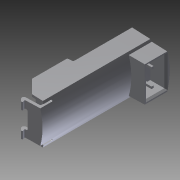
# Autodesk Inventor part: 566716
Saved by Autodesk Inventor 2014 (Build 180170000, 170)
## iProperties
Category: Pneumatics
Company: Autodesk Inc.
Created: 2013-12-30
Part Number: 566716
Catalog Web Link: http://www.festo.com/rep/ko_kr/assets/pdf/VUVG_KR_new.pdf
Vendor: FESTO
Document SubType Name: Modeling
Designer: Autodesk Inc.
Manufacturer: FESTO
Density: 1 g/cm^3
Material: Generic
Appearance: RGB(175.94999939203154,175.94999939203154,175.94999939203154)
Title: 566716 VAVE-L1-1H2-LR
Author: Autodesk Inc.
Autodesk Inventor part; units mm, degrees
sketch "Sketch_23" plane through (0, 0, 0) normal (0, 0, 1) x (1, 0, 0)
  line L0 (-6.5, 4.0058) -> (-3.404, 0.9098)
  line L1 (-3.404, 0.9098) -> (-2.55, 0.8949)
  line L2 (-2.55, 0.8949) -> (-2.55, 0.5951)
  line L3 (-2.55, 0.5951) -> (-4.4413, 0.5621)
  arc A0 (-4.4413, 0.5621) -> (-4.8099, -0.2659) centre (-4.4326, 0.0622) ccw
  line L4 (-4.8099, -0.2659) -> (-4.3557, -0.7885)
  arc A1 (-4.3557, -0.7885) -> (-4.1395, -0.8847) centre (-4.1443, -0.6048) ccw
  line L5 (-4.1395, -0.8847) -> (-3.9988, -0.8823)
  arc A2 (-3.9988, -0.8823) -> (-3.9044, -0.7547) centre (-4.0006, -0.7823) ccw
  line L6 (-3.9044, -0.7547) -> (-4.0447, -0.2655)
  arc A3 (-3.9521, -0.138) -> (-4.0447, -0.2655) centre (-3.9486, -0.2379) ccw
  line L7 (-3.9521, -0.138) -> (0, 0)
  line L8 (0, 0) -> (0, 29)
  line L9 (0, 29) -> (-5.2, 29)
  line L10 (-5.2, 29) -> (-5.2, 15.3866)
  arc A4 (-5.4739, 15.0878) -> (-5.2, 15.3866) centre (-5.5, 15.3866) ccw
  line L11 (-5.4739, 15.0878) -> (-6.2261, 15.022)
  arc A5 (-6.2261, 15.022) -> (-6.5, 14.7231) centre (-6.2, 14.7231) ccw
  line L12 (-6.5, 14.7231) -> (-6.5, 4.0058)
  constraints: 26 end point, 12 point on circle, 6 centre point
extrude "Extrusion1" add sketch "Sketch_23" along normal mid plane 10
sketch "Sketch_1" plane through (0, -5, 0) normal (0, 1, 0) x (1, 0, 0)
  line L0 (-7, 10) -> (-7, -10)
  line L1 (-7, -10) -> (5, -10)
  line L2 (5, -10) -> (5, 10)
  line L3 (5, 10) -> (-7, 10)
  line L4 (-6.5, 4.934) -> (-6.5, -4.934)
  line L5 (-6.5, -4.934) -> (-0.7835, -4.7843)
  arc A0 (-0.7835, -4.7843) -> (-0.7835, 4.7843) centre (-15, 0) ccw
  line L6 (-0.7835, 4.7843) -> (-6.5, 4.934)
  constraints: 14 end point, 2 point on circle, 1 centre point
sketch "Sketch_3" plane through (0, 0, 0) normal (1, 0, 0) x (0, 1, 0)
  line L0 (-3, 5) -> (-3, -5)
  line L1 (-3, -5) -> (1.164, -5)
  line L2 (1.164, -5) -> (1.164, -4.23)
  line L3 (1.164, -4.23) -> (2.722, -4.23)
  arc A0 (2.722, -4.23) -> (2.722, -3.851) centre (2.722, -4.0405) ccw
  line L4 (2.722, -3.851) -> (-1, -3.851)
  line L5 (-1, -3.851) -> (-1, -2.1245)
  line L6 (-1, -2.1245) -> (-0.9, -2.1245)
  line L7 (-0.9, -2.1245) -> (-0.9, 2.1245)
  line L8 (-0.9, 2.1245) -> (-1, 2.1245)
  line L9 (-1, 2.1245) -> (-1, 3.851)
  line L10 (-1, 3.851) -> (2.722, 3.851)
  arc A1 (2.722, 3.851) -> (2.722, 4.23) centre (2.722, 4.0405) ccw
  line L11 (2.722, 4.23) -> (1.164, 4.23)
  line L12 (1.164, 4.23) -> (1.164, 5)
  line L13 (1.164, 5) -> (-3, 5)
  constraints: 28 end point, 4 point on circle, 2 centre point
sketch "Sketch_4" plane through (0, 0, 0) normal (0, 1, 0) x (-1, 0, 0)
  line L0 (6.4, -2.2572) -> (6.4, 2.2572)
  line L1 (6.4, 2.2572) -> (3.6843, 2.1149)
  arc A0 (3.6843, 2.1149) -> (3.4, 1.8153) centre (3.7, 1.8153) ccw
  line L2 (3.4, 1.8153) -> (3.4, -1.8153)
  arc A1 (3.4, -1.8153) -> (3.6843, -2.1149) centre (3.7, -1.8153) ccw
  line L3 (3.6843, -2.1149) -> (6.4, -2.2572)
  constraints: 8 end point, 4 point on circle, 2 centre point
extrude "Extrusion2" cut sketch "Sketch_4" along normal mid plane 2
sketch "Sketch_5" plane through (0, 0, 0) normal (0, 0, 1) x (1, 0, 0)
  line L0 (-15, 0.1264) -> (-15, 3.912)
  line L1 (-15, 3.912) -> (-0.55, 3.912)
  line L2 (-0.55, 3.912) -> (-0.55, 0.9207)
  arc A0 (-0.8395, 0.6209) -> (-0.55, 0.9207) centre (-0.85, 0.9207) ccw
  line L3 (-0.8395, 0.6209) -> (-15, 0.1264)
  line L4 (-15, 0.1264) -> (-15, 3.912)
  constraints: 10 end point, 2 point on circle, 1 centre point
revolve "Revolution1" cut sketch "Sketch_5" angle 60 mid plane about axis through (-15, 0.1264, 0) along (0, 1, 0)
sketch "Sketch_6" plane through (0, 0, 5) normal (0, 0, 1) x (1, 0, 0)
  line L0 (-6.5, 4.0058) -> (-3.404, 0.9098)
  line L1 (-3.404, 0.9098) -> (0, 0.8504)
  line L2 (0, 0.8504) -> (0, 27.33)
  line L3 (0, 27.33) -> (-5.2, 27.33)
  line L4 (-5.2, 27.33) -> (-5.2, 15.3866)
  arc A0 (-5.4739, 15.0878) -> (-5.2, 15.3866) centre (-5.5, 15.3866) ccw
  line L5 (-5.4739, 15.0878) -> (-6.2261, 15.022)
  arc A1 (-6.2261, 15.022) -> (-6.5, 14.7231) centre (-6.2, 14.7231) ccw
  line L6 (-6.5, 14.7231) -> (-6.5, 4.0058)
  constraints: 14 end point, 4 point on circle, 2 centre point
sketch "Sketch_7" plane through (0, 0, -5) normal (0, 0, 1) x (1, 0, 0)
  line L0 (-6.5, 4.0058) -> (-3.404, 0.9098)
  line L1 (-3.404, 0.9098) -> (0, 0.8504)
  line L2 (0, 0.8504) -> (0, 27.33)
  line L3 (0, 27.33) -> (-5.2, 27.33)
  line L4 (-5.2, 27.33) -> (-5.2, 15.3866)
  arc A0 (-5.4739, 15.0878) -> (-5.2, 15.3866) centre (-5.5, 15.3866) ccw
  line L5 (-5.4739, 15.0878) -> (-6.2261, 15.022)
  arc A1 (-6.2261, 15.022) -> (-6.5, 14.7231) centre (-6.2, 14.7231) ccw
  line L6 (-6.5, 14.7231) -> (-6.5, 4.0058)
  constraints: 14 end point, 4 point on circle, 2 centre point
extrude "Extrusion3" cut sketch "Sketch_3" against normal blind 7
extrude "Extrusion4" add sketch "Sketch_6" against normal blind 0.77
extrude "Extrusion5" add sketch "Sketch_7" along normal blind 0.77
sketch "Sketch_12" plane through (0, 0.85, 0) normal (0, 1, 0) x (1, 0, 0)
  line L0 (-6.5, 4.384) -> (-6.5, -4.384)
  line L1 (-6.5, -4.384) -> (-1.2087, -4.2454)
  arc A0 (-1.2087, -4.2454) -> (-1.2087, 4.2454) centre (-15, 0) ccw
  line L2 (-1.2087, 4.2454) -> (-6.5, 4.384)
  constraints: 6 end point, 2 point on circle, 1 centre point
extrude "Extrusion6" cut sketch "Sketch_12" along normal blind 3.062
sketch "Sketch_8" plane through (0, 0, 0) normal (0, 0, 1) x (1, 0, 0)
  arc A0 (-3.603, 3.5593) -> (-3.4556, 3.4093) centre (-3.453, 3.5593) ccw
  line L0 (-3.4556, 3.4093) -> (0, 3.349)
  line L1 (0, 3.349) -> (0, 3.921)
  line L2 (0, 3.921) -> (-3.4556, 3.8607)
  arc A1 (-3.4556, 3.8607) -> (-3.603, 3.7107) centre (-3.453, 3.7107) ccw
  line L3 (-3.603, 3.7107) -> (-3.603, 3.5593)
  constraints: 8 end point, 4 point on circle, 2 centre point
extrude "Extrusion7" add sketch "Sketch_8" along normal mid plane 10
sketch "Sketch_9" plane through (0, 0, -2.693) normal (0, 0, 1) x (1, 0, 0)
  line L0 (-4.154, 0.508) -> (0, 0.508)
  line L1 (0, 0.508) -> (0, 3.405)
  line L2 (0, 3.405) -> (-1.604, 3.405)
  line L3 (-1.604, 3.405) -> (-1.604, 1.1255)
  arc A0 (-1.7693, 0.9285) -> (-1.604, 1.1255) centre (-1.804, 1.1255) ccw
  line L4 (-1.7693, 0.9285) -> (-4.154, 0.508)
  constraints: 10 end point, 2 point on circle, 1 centre point
extrude "Extrusion8" add sketch "Sketch_9" against normal blind 0.512
sketch "Sketch_10" plane through (0, 0, 2.693) normal (0, 0, 1) x (1, 0, 0)
  line L0 (-4.154, 0.508) -> (0, 0.508)
  line L1 (0, 0.508) -> (0, 3.405)
  line L2 (0, 3.405) -> (-1.604, 3.405)
  line L3 (-1.604, 3.405) -> (-1.604, 1.1255)
  arc A0 (-1.7693, 0.9285) -> (-1.604, 1.1255) centre (-1.804, 1.1255) ccw
  line L4 (-1.7693, 0.9285) -> (-4.154, 0.508)
  constraints: 10 end point, 2 point on circle, 1 centre point
extrude "Extrusion9" add sketch "Sketch_10" along normal blind 0.512
sketch "Sketch_15" plane through (0, 2, 0) normal (0, 1, 0) x (1, 0, 0)
  line L0 (-6.5, 4.384) -> (-6.5, -4.384)
  line L1 (-6.5, -4.384) -> (-5.2, -4.35)
  line L2 (-5.2, -4.35) -> (-5.2, 4.35)
  line L3 (-5.2, 4.35) -> (-6.5, 4.384)
  constraints: 8 end point
extrude "Extrusion10" cut sketch "Sketch_15" along normal blind 30
sketch "Sketch_13" plane through (0, 0, 0) normal (0, 0, 1) x (1, 0, 0)
  line L0 (-8.2, 30.398) -> (-8.2, 10.398)
  line L1 (-8.2, 10.398) -> (-6.5, 10.398)
  line L2 (-6.5, 10.398) -> (-6.5, 12.1231)
  arc A0 (-6.2261, 12.422) -> (-6.5, 12.1231) centre (-6.2, 12.1231) ccw
  line L3 (-6.2261, 12.422) -> (-5.4739, 12.4878)
  arc A1 (-5.4739, 12.4878) -> (-5.2, 12.7866) centre (-5.5, 12.7866) ccw
  line L4 (-5.2, 12.7866) -> (-5.2, 30.398)
  line L5 (-5.2, 30.398) -> (-8.2, 30.398)
  constraints: 12 end point, 4 point on circle, 2 centre point
extrude "Extrusion11" cut sketch "Sketch_13" along normal blind 5
extrude "Extrusion12" cut sketch "Sketch_1" along normal blind 35
sketch "Sketch_14" plane through (-5.5, 0, 0) normal (1, 0, 0) x (0, 0, -1)
  line L0 (-4.25, 3.912) -> (4.25, 3.912)
  line L1 (4.25, 3.912) -> (4.25, 29.912)
  line L2 (4.25, 29.912) -> (-4.25, 29.912)
  line L3 (-4.25, 29.912) -> (-4.25, 3.912)
  constraints: 8 end point
extrude "Extrusion13" add sketch "Sketch_14" along normal blind 1.5
sketch "Sketch_17" plane through (-5.5, 0, 0) normal (1, 0, 0) x (0, 0, -1)
  line L0 (-4.25, 25.812) -> (4.25, 25.812)
  line L1 (4.25, 25.812) -> (4.25, 30.812)
  line L2 (4.25, 30.812) -> (-4.25, 30.812)
  line L3 (-4.25, 30.812) -> (-4.25, 25.812)
  constraints: 8 end point
extrude "Extrusion14" cut sketch "Sketch_17" along normal blind 0.3
sketch "Sketch_11" plane through (3.15, 0, 0) normal (1, 0, 0) x (0, 0, -1)
  line L0 (-4.144, 21.162) -> (4.144, 21.162)
  line L1 (4.144, 21.162) -> (4.144, 27.593)
  line L2 (4.144, 27.593) -> (-4.144, 27.593)
  line L3 (-4.144, 27.593) -> (-4.144, 21.162)
  constraints: 8 end point
extrude "Extrusion15" add sketch "Sketch_11" against normal blind 6 draft 1
sketch "Sketch_16" plane through (0, 0, 0) normal (0, 0, 1) x (1, 0, 0)
  line L0 (3.3, 12.312) -> (-5.2, 12.312)
  line L1 (-5.2, 27.312) -> (3.3, 27.0894)
  line L2 (3.3, 27.0894) -> (3.3, 32.312)
  line L3 (3.3, 32.312) -> (-5.2, 32.312)
  line L4 (-5.2, 32.312) -> (-5.2, 27.312)
  constraints: 10 end point
revolve "Revolution2" cut sketch "Sketch_16" angle 40 mid plane about axis through (3.3, 12.312, 0) along (-1, 0, 0)
sketch "Sketch_19" plane through (2.78, 0, 0) normal (1, 0, 0) x (0, 0, -1)
  line L0 (-3.483, 21.83) -> (3.477, 21.83)
  line L1 (3.477, 21.83) -> (3.477, 26.19)
  line L2 (3.477, 26.19) -> (-3.483, 26.19)
  line L3 (-3.483, 26.19) -> (-3.483, 21.83)
  constraints: 8 end point
extrude "Extrusion16" cut sketch "Sketch_19" along normal blind 2 draft 45
sketch "Sketch_20" plane through (2.78, 0, 0) normal (1, 0, 0) x (0, 0, -1)
  line L0 (-3.483, 21.83) -> (3.477, 21.83)
  line L1 (3.477, 21.83) -> (3.477, 26.19)
  line L2 (3.477, 26.19) -> (-3.483, 26.19)
  line L3 (-3.483, 26.19) -> (-3.483, 21.83)
  constraints: 8 end point
extrude "Extrusion17" cut sketch "Sketch_20" against normal blind 3.38
sketch "Sketch_21" plane through (-0.604, 0, 0) normal (1, 0, 0) x (0, 0, -1)
  line L0 (1.75, 23.262) -> (2.25, 23.262)
  line L1 (2.25, 23.262) -> (2.25, 23.762)
  line L2 (2.25, 23.762) -> (1.75, 23.762)
  line L3 (1.75, 23.762) -> (1.75, 23.262)
  constraints: 8 end point
extrude "Extrusion18" add sketch "Sketch_21" along normal blind 3.25
sketch "Sketch_22" plane through (-0.604, 0, 0) normal (1, 0, 0) x (0, 0, -1)
  line L0 (-2.25, 23.262) -> (-1.75, 23.262)
  line L1 (-1.75, 23.262) -> (-1.75, 23.762)
  line L2 (-1.75, 23.762) -> (-2.25, 23.762)
  line L3 (-2.25, 23.762) -> (-2.25, 23.262)
  constraints: 8 end point
extrude "Extrusion19" add sketch "Sketch_22" along normal blind 3.25
sketch "Sketch_2" plane through (-5.5, 0, 0) normal (1, 0, 0) x (0, 0, -1)
  line L0 (1.0745, 9.106) -> (1.0745, 5.255)
  line L1 (1.0745, 5.255) -> (1.9255, 5.255)
  line L2 (1.9255, 5.255) -> (1.9255, 9.106)
  line L3 (1.9255, 9.106) -> (1.0745, 9.106)
  constraints: 8 end point
extrude "Extrusion20" cut sketch "Sketch_2" along normal blind 1.05 draft -1
sketch "Sketch_24" plane through (-5.5, 0, 0) normal (1, 0, 0) x (0, 0, -1)
  line L0 (-1.9255, 9.106) -> (-1.9255, 5.255)
  line L1 (-1.9255, 5.255) -> (-1.0745, 5.255)
  line L2 (-1.0745, 5.255) -> (-1.0745, 9.106)
  line L3 (-1.0745, 9.106) -> (-1.9255, 9.106)
  constraints: 8 end point
extrude "Extrusion21" cut sketch "Sketch_24" along normal blind 1.05 draft -1
sketch "Sketch_25" plane through (0, 0, -1.5) normal (0, 0, 1) x (1, 0, 0)
  line L0 (-3.45, 7.162) -> (-5.5, 7.162)
  line L1 (-5.5, 7.162) -> (-5.5, 8.012)
  line L2 (-5.5, 8.012) -> (-3.45, 7.9404)
  line L3 (-3.45, 7.9404) -> (-3.45, 7.162)
  line L4 (-3.45, 7.162) -> (-5.5, 7.162)
  constraints: 10 end point
revolve "Revolution3" cut sketch "Sketch_25" angle 360 about axis through (-3.45, 7.162, -1.5) along (1, 0, 0)
sketch "Sketch_26" plane through (0, 0, 1.5) normal (0, 0, 1) x (1, 0, 0)
  line L0 (-3.45, 7.162) -> (-5.5, 7.162)
  line L1 (-5.5, 7.162) -> (-5.5, 8.012)
  line L2 (-5.5, 8.012) -> (-3.45, 7.9404)
  line L3 (-3.45, 7.9404) -> (-3.45, 7.162)
  line L4 (-3.45, 7.162) -> (-5.5, 7.162)
  constraints: 10 end point
revolve "Revolution4" cut sketch "Sketch_26" angle 360 about axis through (-3.45, 7.162, 1.5) along (1, 0, 0)
sketch "Sketch_40" plane through (0, 0, 0) normal (0, 0, 1) x (1, 0, 0)
  line L0 (-7.6, 22.574) -> (-2.1, 17.959)
  line L1 (-2.1, 17.959) -> (-2.1, 26.5)
  line L2 (-2.1, 26.5) -> (-0.1, 26.5)
  line L3 (-0.1, 26.5) -> (-0.1, 27.0465)
  arc A0 (-0.1, 27.0465) -> (-0.886, 27.8464) centre (-0.9, 27.0465) ccw
  line L4 (-0.886, 27.8464) -> (-4.704, 27.913)
  line L5 (-4.704, 27.913) -> (-5.5, 27.4073)
  line L6 (-5.5, 27.4073) -> (-6.6349, 27.3677)
  arc A1 (-6.6349, 27.3677) -> (-7.6, 26.3683) centre (-6.6, 26.3683) ccw
  line L7 (-7.6, 26.3683) -> (-7.6, 22.574)
  constraints: 16 end point, 4 point on circle, 2 centre point
extrude "Extrusion22" add sketch "Sketch_40" along normal mid plane 1.722
ref_plane "NEBV_XY" through (-0.004, 23.512, 0) normal (1, 0, 0) x (0, 0, -1)
ref_plane "NEBV_YZ" through (-0.004, 23.512, 0) normal (0, 0, -1) x (0, 1, 0)
ref_plane "NEBV_ZX" through (-0.004, 23.512, 0) normal (0, 1, 0) x (1, 0, 0)
ref_plane "VAVE_XY" through (-4.28, 0, 0) normal (0, -1, 0) x (1, 0, 0)
ref_plane "VAVE_YZ" through (-4.28, 0, 0) normal (1, 0, 0) x (0, 0, 1)
ref_plane "VAVE_ZX" through (-4.28, 0, 0) normal (0, 0, 1) x (0, -1, 0)
body "Solid1"
